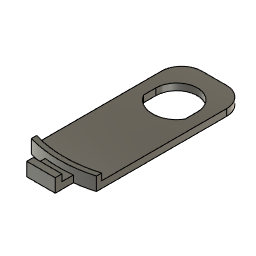
Mount (Autodesk Fusion 360 design; units mm, degrees)
Autodesk Fusion 360 part; units mm, degrees
note: some values were not read from the file. Set by a fixed rule: which sketch regions a step uses.
sketch "Sketch1" plane through (0, 0, 0) normal (0, 0, 1) x (1, 0, 0)
  circle A0 centre (0, 0) radius 7
  dimension "d1" = 14
  constraint coincident A0.centre origin
  measures "d1" diameter of A0
extrude "Extrude1" add sketch "Sketch1" along normal blind 20 makes body 1
sketch "Sketch2" plane through (0, 0, 0) normal (0, 0, 1) x (1, 0, 0)
  line L0 (-7, 0) -> (7, 0)
  line L1 (0, -35) -> (9, -35)
  line L2 (0, -35) -> (-9, -35)
  line L3 (-9, -35) -> (-7, 0)
  line L4 (7, 0) -> (9, -35)
  dimension "d18" = 9
  dimension "d19" = 9
  constraint horizontal L0
  constraint parallel L1 L2
  measures "d18" distance of L1.start L1.end
  measures "d19" distance of L1.start L2.end
extrude "Extrude2" add sketch "Sketch2" along normal blind 2 bodies 1
sketch "Sketch3" plane through (0, 0, 2) normal (0, 0, 1) x (-1, 0, 0)
  arc A0 (7, 0) -> (-7, 0) centre (0, 0) ccw
  line L0 (7, 35) -> (-7, 35)
  line L1 (-7, 35) -> (-7, 31.890001)
  line L2 (-7, 31.890001) -> (7, 31.890001)
  line L3 (7, 31.890001) -> (7, 35)
  line L4 (7, 0) -> (9, 35)
  line L5 (9, 35) -> (-9, 35)
  line L6 (-9, 35) -> (-7, 0)
  constraint horizontal L0
  constraint vertical L1
  constraint horizontal L2
  constraint vertical L3
sketch "Sketch6" plane through (0, 0, 0) normal (0, 0, 1) x (1, 0, 0)
  line L0 (-9, -35.000001) -> (9, -35.000001)
  line L1 (9, -35.000001) -> (9, -38.000001)
  line L2 (9, -38.000001) -> (-9, -38.000001)
  line L3 (-9, -38.000001) -> (-9, -35.000001)
  dimension "d20" = 3
  constraint horizontal L0
  constraint vertical L1
  constraint horizontal L2
  constraint vertical L3
extrude "Extrude4" add sketch "Sketch6" along normal blind 20 bodies 1
sketch "Sketch7" plane through (0, -38.000001, 0) normal (0, -1, 0) x (1, 0, 0)
  line L0 (-9, 0) -> (9, 0)
  line L1 (9, 0) -> (9, 20)
  line L2 (9, 20) -> (-9, 20)
  line L3 (-9, 20) -> (-9, 0)
  line L4 (-7.5, 17.5) -> (7.5, 17.5)
  line L5 (7.5, 17.5) -> (7.5, 14.5)
  line L6 (7.5, 14.5) -> (-7.5, 14.5)
  line L7 (-7.5, 14.5) -> (-7.5, 17.5)
  line L8 (-7.5, 11.4) -> (7.5, 11.4)
  line L9 (7.5, 11.4) -> (7.5, 8.4)
  line L10 (7.5, 8.4) -> (-7.5, 8.4)
  line L11 (-7.5, 8.4) -> (-7.5, 11.4)
  line L12 (-7.5, 5.3) -> (7.5, 5.3)
  line L13 (7.5, 5.3) -> (7.5, 2.3)
  line L14 (7.5, 2.3) -> (-7.5, 2.3)
  line L15 (-7.5, 2.3) -> (-7.5, 5.3)
  dimension "d23" = 15
  dimension "d24" = 3
  dimension "d25" = 1.5
  dimension "d26" = 1.5
  dimension "d27" = 15
  dimension "d28" = 3
  dimension "d29" = 15
  dimension "d30" = 3
  dimension "d31" = 3.1
  dimension "d32" = 3.1
  dimension "d33" = 2.5
  dimension "d34" = 2.3
  constraint horizontal L4
  constraint vertical L5
  constraint horizontal L6
  constraint vertical L7
  constraint horizontal L8
  constraint vertical L9
  constraint horizontal L10
  constraint vertical L11
  constraint horizontal L12
  constraint vertical L13
  constraint horizontal L14
  constraint vertical L15
  measures "d23" distance of L4.start L4.end
  measures "d24" distance of L4.start L6.end
  measures "d25" distance of L3 L7
  measures "d26" distance of L1 L5
  measures "d27" distance of L8.start L8.end
  measures "d28" distance of L8.start L10.end
  measures "d29" distance of L12.start L12.end
  measures "d30" distance of L12.start L14.end
  measures "d31" distance of L6 L8
  measures "d32" distance of L10 L12
  measures "d33" distance of L2 L4
  measures "d34" distance of L0 L14
extrude "Extrude5" add sketch "Sketch7" along normal blind 15.5 contours L4 L5 L6 L7 | L8 L9 L10 L11 | L12 L13 L14 L15 picked at (-2.5, 16.5) picked at (-2.5, 10.4) picked at (-2.5, 4.3) bodies 1
sketch "Sketch8" plane through (0, 0, 17.5) normal (0, 0, 1) x (-1, 0, 0)
  line L0 (-7.5, 38.000001) -> (7.5, 38.000001)
  line L1 (7.5, 38.000001) -> (7.5, 53.500001)
  line L2 (7.5, 53.500001) -> (-7.5, 53.500001)
  line L3 (-7.5, 53.500001) -> (-7.5, 38.000001)
  circle A0 centre (0, 46.000001) radius 2.8
  line L4 (9, 38.000001) -> (-9, 38.000001)
  arc A1 (7.5, 46.000001) -> (-7.5, 45.998582) centre (0, 46.000001) ccw
  line L5 (7.5, 46.000001) -> (9, 46.000001)
  line L6 (9, 46.000001) -> (9, 55.000001)
  line L7 (9, 55.000001) -> (-9, 55.000001)
  line L8 (-9, 55.000001) -> (-9, 46.000001)
  line L9 (-9, 46.000001) -> (-7.5, 45.998582)
  dimension "d37" = 5.6
  dimension "d38" = 8
  dimension "d39" = 7.5
  dimension "d40" = 7.5
  constraint concentric A0 A1
  constraint perpendicular L1 L5
  constraint perpendicular L5 L6
  constraint perpendicular L6 L7
  constraint perpendicular L7 L8
  measures "d37" diameter of A0
extrude "Extrude6" cut sketch "Sketch8" against normal blind 21 contours L1 L2 L3 L5 L6 L7 L8 L9 | L1 L2 A1 | A0 picked at (0, 54.500001) picked at (6.026526, 52.026526) picked at (-0.771156, 46.525766) bodies 1
sketch "Sketch10" plane through (0, 0, 20) normal (0, 0, 1) x (-1, 0, 0)
  circle A0 centre (0, 0) radius 7
  circle A1 centre (0, 0) radius 6
  dimension "d45" = 12
  constraint coincident A0.centre A1.centre
  measures "d45" diameter of A1
extrude "Extrude8" add sketch "Sketch10" along normal blind 2.2 contours A1 picked at (-0.9566, -0.291426) bodies 1
sketch "Sketch13" plane through (0, -38.000001, 0) normal (0, -1, 0) x (1, 0, 0)
  line L0 (-7.5, 2.3) -> (-7.5, 5.3)
  line L1 (-7.5, 5.3) -> (7.5, 5.3)
  line L2 (7.5, 5.3) -> (7.5, 2.3)
  line L3 (7.5, 2.3) -> (-7.5, 2.3)
  line L4 (-7.5, 8.4) -> (-7.5, 11.4)
  line L5 (-7.5, 11.4) -> (7.5, 11.4)
  line L6 (7.5, 11.4) -> (7.5, 8.4)
  line L7 (7.5, 8.4) -> (-7.5, 8.4)
  line L8 (-7.5, 14.5) -> (-7.5, 17.5)
  line L9 (-7.5, 17.5) -> (7.5, 17.5)
  line L10 (7.5, 17.5) -> (7.5, 14.5)
  line L11 (7.5, 14.5) -> (-7.5, 14.5)
  line L12 (-9, 0) -> (9, 0)
  line L13 (9, 0) -> (9, 20)
  line L14 (9, 20) -> (-9, 20)
  line L15 (-9, 20) -> (-9, 0)
  line L16 (-9, 20) -> (-9, 22)
  line L17 (-9, 22) -> (-9, 24)
  line L18 (4, 21) -> (4, 22)
  line L19 (-4.5, 22) -> (-4.5, 20)
  line L20 (9, 25) -> (-9, 25)
  line L21 (-9, 25) -> (-9, 24)
  line L22 (4, 22) -> (4, 22.2)
  line L23 (4, 22.2) -> (-4.5, 22.2)
  line L24 (-4.5, 22.2) -> (-4.5, 22)
  line L25 (4, 21) -> (9, 21)
  line L26 (9, 21) -> (9, 25)
  constraint coincident L14.end L15.start
  constraint perpendicular L14 L16
  constraint perpendicular L14 L17
  constraint horizontal L20
  constraint vertical L21
  constraint vertical L22
  constraint horizontal L23
  constraint vertical L24
  constraint perpendicular L18 L25
extrude "Extrude11" add sketch "Sketch13" against normal blind 3 contours L14 L16 L17 L18 L19 L20 L21 L22 L23 L24 L25 L26 picked at (-1.5, 24.066667) bodies 1
sketch "Sketch15" plane through (0, 0, 0) normal (0, 0, 1) x (1, 0, 0)
  line L0 (50.300001, 8.7) -> (57.700001, 8.7)
  line L1 (63.700001, 2.7) -> (63.700001, -15.104525)
  line L2 (44.300001, -15.104525) -> (44.300001, 2.7)
  line L3 (54.000001, -15.104525) -> (54.000001, -44.000001)
  line L4 (54.000001, -37.5) -> (49.500001, -37.5)
  line L5 (54.000001, -37.5) -> (58.000001, -37.5)
  line L6 (44.300001, -15.104525) -> (44.300001, -36.129005)
  line L7 (63.700001, -15.104525) -> (63.700001, -36.129005)
  line L8 (49.500001, -37.5) -> (58.000001, -37.5)
  line L9 (58.000001, -37.5) -> (58.000001, -39.5)
  line L10 (58.000001, -39.5) -> (49.500001, -39.5)
  line L11 (49.500001, -39.5) -> (49.500001, -37.5)
  arc A0 (44.300001, -36.129005) -> (63.700001, -36.129005) centre (54.000001, -2.5) ccw
  arc A1 (50.300001, 8.7) -> (44.300001, 2.7) centre (50.300001, 2.7) ccw
  arc A2 (63.700001, 2.7) -> (57.700001, 8.7) centre (57.700001, 2.7) ccw
  arc A3 (44.300001, -34.564934) -> (63.700001, -34.564934) centre (54.000001, -2.5) ccw
  line L12 (49.500001, -37.5) -> (49.500001, -37.209509)
  line L13 (58.000001, -37.5) -> (58.000001, -37.270677)
  line L14 (53.500001, -2.5) -> (54.500001, -2.5)
  line L15 (54.000001, -2.994277) -> (54.000001, -2)
  line L16 (47.800001, -6.160601) -> (47.800001, -2.5)
  arc A4 (60.200001, -2.5) -> (47.800001, -2.5) centre (54.000001, -2.5) ccw
  line L17 (60.200001, -2.5) -> (60.200001, -6.160601)
  arc A5 (47.800001, -6.160601) -> (60.200001, -6.160601) centre (54.000001, -2.5) ccw
  dimension "d85" = 4.5
  dimension "d86" = 4
  dimension "d87" = 2
  dimension "d88" = 6
  dimension "d89" = 6
  constraint horizontal L0
  constraint vertical L1
  constraint vertical L2
  constraint perpendicular L3 L4
  constraint perpendicular L3 L5
  constraint perpendicular L4 L6
  constraint perpendicular L5 L7
  constraint horizontal L8
  constraint vertical L9
  constraint horizontal L10
  constraint vertical L11
  constraint tangent L2 A1
  constraint tangent L0 A1
  constraint tangent L0 A2
  constraint tangent L1 A2
  constraint perpendicular L3 L14
  constraint perpendicular L14 L15
  measures "d88" radius of A1
  measures "d89" radius of A2
extrude "Extrude12" add sketch "Sketch15" along normal blind 2 separate body makes body 2
sketch "Sketch16" plane through (0, 0, 2) normal (0, 0, 1) x (-1, 0, 0)
  line L0 (-58.000001, 39.5) -> (-58.000001, 37.270677)
  arc A0 (-58.000001, 37.270677) -> (-63.700001, 36.129005) centre (-54.000001, 2.5) ccw
  line L1 (-63.700001, 36.129005) -> (-63.700001, -2.7)
  arc A1 (-63.700001, -2.7) -> (-57.700001, -8.7) centre (-57.700001, -2.7) ccw
  line L2 (-57.700001, -8.7) -> (-50.300001, -8.7)
  arc A2 (-50.300001, -8.7) -> (-44.300001, -2.7) centre (-50.300001, -2.7) ccw
  line L3 (-44.300001, -2.7) -> (-44.300001, 36.129005)
  arc A3 (-44.300001, 36.129005) -> (-49.500001, 37.209509) centre (-54.000001, 2.5) ccw
  line L4 (-49.500001, 37.209509) -> (-49.500001, 39.5)
  line L5 (-49.500001, 39.5) -> (-58.000001, 39.5)
  arc A4 (-44.300001, 34.564934) -> (-63.700001, 34.564934) centre (-54.000001, 2.5) ccw
  arc A5 (-44.300001, 36.129005) -> (-63.700001, 36.129005) centre (-54.000001, 2.5) ccw
  line L6 (-44.300001, 34.564934) -> (-44.300001, 36.129005)
  line L7 (-63.700001, 34.564934) -> (-63.700001, 36.129005)
  arc A6 (-60.200001, 2.5) -> (-47.800001, 2.5) centre (-54.000001, 2.5) ccw
  line L8 (-60.200001, 2.5) -> (-60.200001, 6.160601)
  arc A7 (-47.800001, 6.160601) -> (-60.200001, 6.160601) centre (-54.000001, 2.5) ccw
  line L9 (-47.800001, 6.160601) -> (-47.800001, 2.5)
  dimension "d93" = 67
  constraint concentric A0 A4
  constraint concentric A0 A5
  measures "d93" diameter of A4
extrude "Extrude13" add sketch "Sketch16" along normal blind 2 contours A0 L1 L3 A3 A4 A5 L6 L7 picked at (-61.474957, 35.60632) bodies 2
sketch "Sketch17" plane through (0, -39.5, 0) normal (0, -1, 0) x (1, 0, 0)
  line L0 (49.500001, 0) -> (58.000001, 0)
  line L1 (58.000001, 0) -> (58.000001, 2)
  line L2 (58.000001, 2) -> (49.500001, 2)
  line L3 (49.500001, 2) -> (49.500001, 0)
  line L4 (49.500001, 2) -> (58.000001, 2)
  line L5 (58.000001, 2) -> (58.000001, 0)
  line L6 (58.000001, 0) -> (49.500001, 0)
  line L7 (49.500001, 0) -> (49.500001, 2)
  constraint horizontal L4
  constraint vertical L5
  constraint horizontal L6
  constraint vertical L7
extrude "Extrude14" add sketch "Sketch17" along normal blind 3.2 bodies 2
sketch "Sketch18" plane through (0, 0, 2) normal (0, 0, 1) x (-1, 0, 0)
  arc A0 (-49.500001, 37.209509) -> (-58.000001, 37.270677) centre (-54.000001, 2.5) ccw
  line L0 (-49.500001, 37.209509) -> (-49.500001, 42.7)
  line L1 (-49.500001, 42.7) -> (-58.000001, 42.7)
  line L2 (-58.000001, 42.7) -> (-58.000001, 37.270677)
  line L3 (-49.500001, 42.7) -> (-58.000001, 42.7)
  line L4 (-58.000001, 42.7) -> (-58.000001, 40.7)
  line L5 (-58.000001, 40.7) -> (-49.500001, 40.7)
  line L6 (-49.500001, 40.7) -> (-49.500001, 42.7)
  dimension "d98" = 2
  constraint horizontal L3
  constraint vertical L4
  constraint horizontal L5
  constraint vertical L6
extrude "Extrude15" add sketch "Sketch18" along normal blind 2 contours L0 L1 L2 L3 L4 L5 L6 picked at (-52.333334, 42.033333) bodies 2
copy_body "Body->Comp3" bodies 2 removing the originals makes body 3 in component "Component"
copy_body "Body->Comp4" bodies 1 removing the originals makes body 4 in component "Component'"
extrude "Extrude2'" add 1 faces at (-0.069748, -39.735944, 2.3) along direction (0, 0, -1) up to surface (2.3 mm away) on bodies 4 bodies 4 in component "Component'"
sketch "Sketch22" plane through (0, 0, 22.2) normal (0, 0, 1) x (-1, 0, 0)
  circle A0 centre (0, 0) radius 6
  circle A1 centre (0, 0) radius 7
  line L0 (6, 0) -> (-6, 0)
  line L1 (-6, 0) -> (-6, -7)
  line L2 (-6, -7) -> (6, -7)
  line L3 (6, -7) -> (6, 0)
  constraint coincident A0.centre A1.centre
  constraint horizontal L0
  constraint vertical L1
  constraint horizontal L2
  constraint vertical L3
  constraint coincident A0 L0.start
extrude "Extrude6'" add sketch "Sketch22" along normal blind 2 contours A0 L0 | A0 A1 L1 L3 | A0 L0 picked at (1.824276, 1.165852) picked at (-0.491456, -6.635875) picked at (-1.466104, -1.360345) bodies 4 in component "Component'"
component "Component" placed x (1, 0, 0) y (0, 1, 0) z (0, 0, 1) at (0, 0, 0)
component "Component'" placed x (1, 0, 0) y (0, 1, 0) z (0, 0, 1) at (0, 0, 0)
